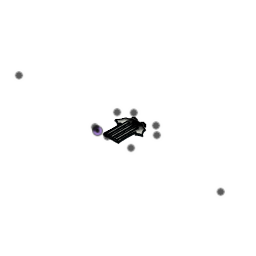
LLAVERO (Autodesk Fusion 360 design; units mm, degrees)
Autodesk Fusion 360 part; units mm, degrees
sketch "Boceto1" plane through (0, 0, 0) normal (0, 0, 1) x (1, 0, 0)
  spline S0 degree 5 poles (17, 50) (17.32, 49.4691) (17.96, 48.4536) (18.92, 47.0694) (20.2, 45.5067) (21.8, 44.0566) (23.4, 43.1548) (25, 42.846) (26.6, 43.1548) (28.2, 44.0566) (29.8, 45.5067) (31.08, 47.0694) (32.04, 48.4536) (32.68, 49.4691) (33, 50) knots 0 0 0 0 0 0 0.1 0.2 0.3 0.4 0.5 0.6 0.7 0.8 0.9 1 1 1 1 1 1
  line L0 (25, 43) -> (25, 0) construction
  arc A0 (7, 45) -> (17, 50) centre (4.4264, 62.6472) ccw
  arc A1 (0, 33) -> (7, 45) centre (-11.8333, 47.9444) ccw
  arc A2 (8.6345, 29.0047) -> (0, 33) centre (-8.4336, 3.4454) ccw
  line L1 (8.6345, 29.0047) -> (11.4903, 32.3049)
  arc A3 (11.4903, 0) -> (11.4903, 32.3049) centre (-162.0039, 16.1524) ccw
  arc A4 (33, 50) -> (43, 45) centre (45.5736, 62.6472) ccw
  arc A5 (43, 45) -> (50, 33) centre (61.8333, 47.9444) ccw
  arc A6 (50, 33) -> (41.3655, 29.0047) centre (58.4336, 3.4454) ccw
  line L2 (41.3655, 29.0047) -> (38.5097, 32.3049)
  arc A7 (38.5097, 32.3049) -> (38.5097, 0) centre (212.0039, 16.1524) ccw
  line L3 (17, 50) -> (33, 50)
  circle A8 centre (25, 47) radius 1.5
  line L4 (18, 0) -> (15, 0)
  line L5 (19, 41) -> (19, 0)
  line L6 (19, 0) -> (15, 0)
  line L7 (15, 0) -> (15, 41)
  line L8 (23, 41) -> (23, 0)
  line L9 (23, 0) -> (27, 0)
  line L10 (27, 0) -> (27, 41)
  line L11 (31, 41) -> (31, 0)
  line L12 (31, 0) -> (35, 0)
  line L13 (35, 0) -> (35, 41)
  arc A9 (23, 41) -> (27, 41) centre (25, 44.75) ccw
  arc A10 (15, 41) -> (19, 41) centre (17, 44.75) ccw
  arc A11 (31, 41) -> (35, 41) centre (33, 44.75) ccw
  line L14 (11.4903, 0) -> (38.5097, 0)
  point P0 (25, 43)
  dimension "d10" = 3
  dimension "d11" = 4
  dimension "d12" = 4
  dimension "d15" = 4
  dimension "d16" = 4
  dimension "d17" = 4
  dimension "d18" = 174.2445
  dimension "d19" = 19.0621
  dimension "d20" = 30.7343
  dimension "d21" = 17.8339
  dimension "d22" = 4.25
  dimension "d23" = 2
  dimension "d24" = 1
  dimension "d25" = 8.4336
  dimension "d26" = 3.4454
  dimension "d27" = 33.4336
  dimension "d28" = 46.5546
  dimension "d29" = 43.5546
  dimension "d30" = 39.5546
  dimension "d31" = 40.871
  dimension "d32" = 220.4376
  dimension "d33" = 70.267
  dimension "d34" = 59.2018
  dimension "d35" = 49.7991
  constraint coincident P0 L0.start
  constraint symmetric S0.start L0 S0.end
  constraint symmetric A0.start L0 A4.end
  constraint symmetric A1.start L0 A5.end
  constraint symmetric L0 A0 A4
  constraint symmetric L0 A1 A5
  constraint symmetric L0 A2.start A6.end
  constraint symmetric L0 A2 A6
  constraint symmetric L0 L1.end L2.end
  constraint symmetric L0 A3.start A7.end
  constraint symmetric L0 A3 A7
  constraint horizontal L3
  constraint perpendicular L5 L6
  constraint perpendicular L8 L9
  constraint perpendicular L11 L12
  constraint perpendicular L13 L14
  constraint perpendicular L4 L7
  constraint perpendicular L9 L10
  constraint perpendicular L12 L13
  constraint parallel L4 L6
  constraint collinear L4 L6
  constraint collinear L12 L14
  constraint coincident L4.end L6.end
  constraint coincident S0.end A4.start
  constraint coincident L0.end L14
  constraint coincident L4.end L14
  constraint coincident L5.end L14
  constraint coincident L8.end L14
  constraint coincident L9.end L14
  constraint coincident L11.end L14
  constraint coincident S0 P0
  constraint vertical S0.start A10.centre
  constraint vertical P0 A9.centre
  constraint vertical P0 A8.centre
  constraint vertical S0.end A11.centre
  constraint horizontal L7.end L10.end
  constraint horizontal L7.end L8.start
  constraint horizontal A9.centre A10.centre
  constraint horizontal L7.end L13.end
  constraint horizontal L7.end L11.start
  constraint horizontal A10.centre A11.centre
  constraint vertical origin A1.start
  constraint horizontal origin A3.start
  measures "d10" diameter of A8
  measures "d11" distance of L7.end L5.start
  measures "d12" distance of L5.end L4.end
  measures "d15" distance of L8.end L9.end
  measures "d16" distance of L10.end L11.start
  measures "d17" distance of L11.end L12.end
  measures "d18" radius of A7
  measures "d19" radius of A5
  measures "d20" radius of A6
  measures "d21" radius of A4
  measures "d22" radius of A10
  measures "d23" distance of S0.start L5
  measures "d24" horizontal distance of L4.start A10.centre
  measures "d25" horizontal distance of origin A2.centre
  measures "d26" vertical distance of origin A2.centre
  measures "d27" distance of L0 A2.centre
  measures "d28" distance of A2.centre L3
  measures "d29" vertical distance of A2.centre A8.centre
  measures "d30" vertical distance of P0 A2.centre
  measures "d31" angle of L2 L13
  measures "d32" horizontal distance of A2.centre A7.centre
  measures "d33" horizontal distance of A2.centre A5.centre
  measures "d34" vertical distance of A0.centre A2.centre
  measures "d35" horizontal distance of A2.centre A6.end
extrude "Extruir1" add sketch "Boceto1" along normal blind 2 contours S0 A0 A1 A2 L1 A3 A4 A5 A6 L2 A7 L5 L7 L8 L10 L11 L13 A9 A10 A11 L14
extrude "Extruir2" add sketch "Boceto1" along normal blind 3 contours L4 L5 L6 L7 A10 L14
extrude "Extruir3" add sketch "Boceto1" along normal blind 3 contours L8 L9 L10 A9 L14
extrude "Extruir4" add sketch "Boceto1" along normal blind 3 contours L11 L12 L13 A11 L14
extrude "Extruir5" add sketch "Boceto1" along normal blind 1.5 contours S0 L3
